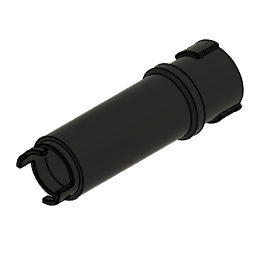
proximal_needle_cover_rev_D_v2 (Autodesk Fusion 360 design; units mm, degrees)
Autodesk Fusion 360 part; units mm, degrees
sketch "Sketch1" plane through (0, 0, 0) normal (0, 1, 0) x (1, 0, 0)
  circle A0 centre (0, 0) radius 10.4
  circle A1 centre (0, 0) radius 12
  circle A2 centre (0, 0) radius 8.8
  dimension "d1" = 20.8
  dimension "d2" = 24
  dimension "d3" = 17.6
  constraint coincident A0.centre A1.centre
  measures "d1" diameter of A0
  measures "d2" diameter of A1
  measures "d3" diameter of A2
extrude "Extrude1" add sketch "Sketch1" along normal blind 75 and the other way blind 2.5 contours A1
extrude "Extrude2" add sketch "Sketch1" against normal blind 5.5 contours A0
ref_plane "WorkPlane1" through (0, -5.6, 0) normal (0, 1, 0) x (0, 0, 1)
sketch "Sketch2" plane through (0, -5.6, 0) normal (0, 1, 0) x (1, 0, 0)
sketch "Sketch3" plane through (0, -5.5, 0) normal (0, -1, 0) x (1, 0, 0)
  circle A0 centre (0, 0) radius 8.8
  circle A1 centre (0, 0) radius 10.4
  circle A2 centre (0, 0) radius 10.4
  circle A3 centre (0, 0) radius 8.8
  line L0 (0, 8.8) -> (0, 10.4)
  line L1 (0, -8.8) -> (0, -10.4)
  line L2 (8.7946, -0.3071) -> (10.3937, -0.363)
  line L3 (-8.7946, 0.3071) -> (-10.3937, 0.363)
  line L4 (-8.7946, 0.3071) -> (8.7946, -0.3071) construction
  line L5 (-7.4628, 4.6633) -> (7.4628, -4.6633) construction
  line L6 (-7.4628, 4.6633) -> (-8.8197, 5.5112)
  line L7 (7.4628, -4.6633) -> (8.8197, -5.5112)
  dimension "d11" = 88
  dimension "d12" = 30
  constraint coincident A3 L0.start
  constraint coincident A1 L0.end
  constraint vertical L0
  constraint coincident A0 L1.start
  constraint coincident A2 L1.end
  constraint parallel L0 L1
  constraint coincident A3 L2.start
  constraint coincident A2 L2.end
  constraint coincident A3 L3.start
  constraint coincident A2 L3.end
  constraint parallel L2 L3
  constraint vertical L0.start A0.centre
  constraint vertical L1.start A0.centre
  constraint coincident A0.centre L4
  constraint collinear L3 L4
  constraint coincident A3 L5.start
  constraint coincident A0.centre L5
  constraint coincident A0 L5.end
  constraint coincident A2 L6.end
  constraint parallel L5 L6
  constraint coincident A2 L7.end
  constraint parallel L5 L7
  measures "d11" angle of L0 L3
  measures "d12" angle of L3 L6
extrude "Extrude3" add sketch "Sketch3" along normal blind 7 contours A0 A1 A2 A3 L2 L7 | A0 A1 A2 A3 L3 L6
extrude "Extrude4" add sketch "Sketch3" along normal blind 2.8 from surface at 2.1 contours A0 A1 A2 A3 L0 L6 | A0 A1 A2 A3 L1 L7
sketch "Sketch4" plane through (0, 75, 0) normal (0, 1, 0) x (-1, 0, 0)
  circle A0 centre (0, 0) radius 10.4
  circle A1 centre (0, 0) radius 12
  circle A2 centre (0, 0) radius 11.2
  dimension "d24" = 22.4
  constraint concentric A0 A2
  measures "d24" diameter of A2
extrude "Extrude5" cut sketch "Sketch4" against normal up to surface (75 mm away) contours A2
fillet "Fillet1" radius 0.5 16 edges at (-8.1413, -5.5, 5.0872) (-8.1413, -7.6, 5.0872) (8.1413, -7.6, -5.0872) (8.1413, -5.5, -5.0872) (9.5942, -5.5, -0.335) (-9.5942, -5.5, 0.335) (-8.1413, -10.4, 5.0872) (8.1413, -10.4, -5.0872) (9.5942, -12.5, -0.335) (8.1413, -12.5, -5.0872) (0, -10.4, 9.6) (0, -7.6, 9.6) (-8.1413, -12.5, 5.0872) (-9.5942, -12.5, 0.335) (0, -10.4, -9.6) (0, -7.6, -9.6)
fillet "Fillet2" radius 0.25 64 edges at (8.8197, -11.45, -5.5112) (8.8965, -12.3536, -5.3864) (9.9456, -12.5, -3.0407) (10.3875, -12.3536, -0.5093) (10.3937, -9, -0.363) (10.3977, -5.6464, -0.2165) (3.0407, -5.5, 9.9456) (-8.7412, -5.6464, 5.6349) (-8.8197, -6.55, 5.5112) (-8.7412, -7.4536, 5.6349) (-5.042, -7.6, 9.096) (-0.1465, -7.7464, 10.399) (0, -9, 10.4) (-0.1465, -10.2536, 10.399) (-5.042, -10.4, 9.096) (-8.7412, -10.5464, 5.6349) (-8.8197, -11.45, 5.5112) (-8.8965, -12.3536, 5.3864) (-9.9456, -12.5, 3.0407) (-10.3875, -12.3536, 0.5093) (-10.3937, -9, 0.363) (-10.3977, -5.6464, 0.2165) (-3.0407, -5.5, -9.9456) (8.7412, -5.6464, -5.6349) (8.8197, -6.55, -5.5112) (8.7412, -7.4536, -5.6349) (5.042, -7.6, -9.096) (0.1465, -7.7464, -10.399) (0, -9, -10.4) (0.1465, -10.2536, -10.399) (5.042, -10.4, -9.096) (8.7412, -10.5464, -5.6349) (8.7946, -9, -0.3071) (8.7883, -12.3536, -0.4535) (8.4155, -12.5, -2.5729) (7.5394, -12.3536, -4.5384) (7.4628, -11.45, -4.6633) (7.3841, -10.5464, -4.7869) (4.2663, -10.4, -7.6967) (0.1465, -10.2536, -8.7988) (0, -9, -8.8) (0.1465, -7.7464, -8.7988) (4.2663, -7.6, -7.6967) (7.3841, -7.4536, -4.7869) (7.4628, -6.55, -4.6633) (7.3841, -5.6464, -4.7869) (-2.5729, -5.5, -8.4155) (-8.7985, -5.6464, 0.1606) (-8.7946, -9, 0.3071) (-8.7883, -12.3536, 0.4535) (-8.4155, -12.5, 2.5729) (-7.5394, -12.3536, 4.5384) (-7.4628, -11.45, 4.6633) (-7.3841, -10.5464, 4.7869) (-4.2663, -10.4, 7.6967) (-0.1465, -10.2536, 8.7988) (0, -9, 8.8) (-0.1465, -7.7464, 8.7988) (-4.2663, -7.6, 7.6967) (-7.3841, -7.4536, 4.7869) (-7.4628, -6.55, 4.6633) (-7.3841, -5.6464, 4.7869) (2.5729, -5.5, 8.4155) (8.7985, -5.6464, -0.1606)
fillet "Fillet3" [suppressed]
chamfer "Chamfer2" [suppressed]
sketch "Sketch5" plane through (0, 75, 0) normal (0, 1, 0) x (-1, 0, 0)
  circle A0 centre (0, 0) radius 12
  circle A1 centre (0, 0) radius 13.5
  line L0 (11.4486, 7.1539) -> (10.1766, 6.359)
  line L1 (-10.1766, -6.359) -> (-11.4486, -7.1539)
  line L2 (0, 12) -> (0, 13.5)
  line L3 (0, -12) -> (0, -13.5)
  line L4 (10.1766, 6.359) -> (-10.1766, -6.359) construction
  line L5 (0, 12) -> (0, -12) construction
  dimension "d29" = 27
  dimension "d35" = 58
  constraint coincident A1 L0.start
  constraint coincident A0 L0.end
  constraint coincident A0 L1.start
  constraint coincident A1 L1.end
  constraint coincident A0 L2.start
  constraint coincident A1 L2.end
  constraint coincident A0 L3.start
  constraint coincident A1 L3.end
  constraint coincident A0.centre L5
  constraint coincident A0.centre L4
  constraint coincident A0.centre A1.centre
  constraint vertical L5
  constraint collinear L0 L4
  constraint collinear L1 L4
  constraint collinear L2 L5
  constraint collinear L3 L5
  measures "d29" diameter of A1
  measures "d35" angle of L4 L5
extrude "Extrude6" add sketch "Sketch5" against normal blind 25 contours A0 A1 L0 L3 | A0 A1 L0 L2 | A0 A1 L1 L3 | A0 A1 L1 L2
extrude "Extrude7" cut sketch "Sketch5" against normal blind 10.1 from surface at -9.9 contours A0 A1 L0 L2 | A0 A1 L1 L3
extrude "Extrude8" cut sketch "Sketch5" against normal blind 20 contours A0 A1 L0 L3 | A0 A1 L1 L2
draft "Draft1" angle 1.75 neutral plane through (0, 75, 0) pull (0, 1, 0) 1 faces at (-11.1861, 25, -0.5583)
fillet "Fillet4" radius 0.5 6 edges at (-11.4486, 70.05, 7.1539) (-6.5449, 65.1, 11.8074) (0, 70.05, 13.5) (0, 70.05, -13.5) (6.5449, 65.1, -11.8074) (11.4486, 70.05, -7.1539)
fillet "Fillet4" radius 0.5 4 edges at (0, 65.1, 12.75) (-10.8126, 65.1, 6.7565) (10.8126, 65.1, -6.7565) (0, 65.1, -12.75)
chamfer "Chamfer1" distance 1.5 angle 45 1 edges at (12.5864, 50, 4.8818)
